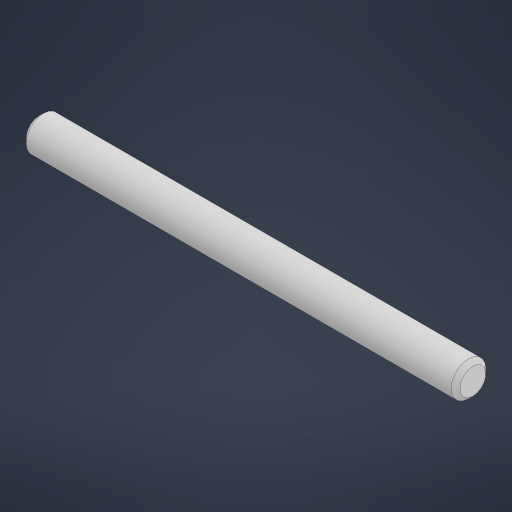
# Autodesk Inventor part: Część28
Saved by Autodesk Inventor 2023 (Build 270158000, 158)
## iProperties
Created: 2023-05-09
Part Number: Część28
Material: Ogólny
Document SubType Name: Modeling
Designer: Adam
Density: 1 g/cm^3
Appearance: Domyślna
Author: Adam
Autodesk Inventor part; units mm, degrees
ref_plane "YZ Plane" through (0, 0, 0) normal (1, 0, 0) x (0, 1, 0)
ref_plane "XZ Plane" through (0, 0, 0) normal (0, 1, 0) x (-1, 0, 0)
ref_plane "XY Plane" through (0, 0, 0) normal (0, 0, 1) x (1, 0, 0)
sketch "Szkic1" plane through (0, 0, 0) normal (0, 0, 1) x (1, 0, 0)
  point P0 (0, 0)
sketch "Szkic2" plane through (0, 0, 0) normal (0, 0, 1) x (1, 0, 0)
  line L0 (-25, 0) -> (25, 0)
  line L1 (25, 0) -> (25, 2)
  line L2 (25, 2) -> (-25, 2)
  line L3 (-25, 2) -> (-25, 0)
  point P0 (0, 0)
  point P1 (0, 1)
  dimension "d0" = 50
  dimension "d1" = 2
  constraints: 8 end point, 2 parallel, 1 horizontal, 1 perpendicular
  measures "d0" distance of L2.end L1.end
  measures "d1" distance of L1.end L0.end
revolve "Obrót1" add sketch "Szkic2" angle 360 about axis through (-25, 0, 0) along (1, 0, 0)
chamfer "Faza1" distance 0.5 angle 45 1 edges at (25, -2, 0) measured on face at (25, 0.0679, 1.2634)
chamfer "Faza2" distance 0.5 angle 45 1 edges at (-25, -2, 0) measured on face at (-25, 0.6473, -0.1595)
